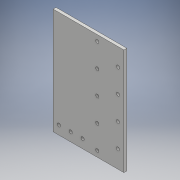
# Autodesk Inventor part: GanrtyPlatev2
Saved by Autodesk Inventor 2017 (Build 210142000, 142)
## iProperties
Created: 2017-03-07
Part Number: GanrtyPlatev2
Material: Generic
Document SubType Name: Modeling
Designer: umr
Density: 1 g/cm^3
Appearance: Default
Author: umr
Autodesk Inventor part; units mm, degrees
ref_plane "YZ Plane" through (0, 0, 0) normal (1, 0, 0) x (0, 1, 0)
ref_plane "XZ Plane" through (0, 0, 0) normal (0, 1, 0) x (-1, 0, 0)
ref_plane "XY Plane" through (0, 0, 0) normal (0, 0, 1) x (1, 0, 0)
sketch "Sketch1" plane through (0, 0, 0) normal (0, 1, 0) x (-1, 0, 0)
  line L0 (0, 0) -> (120, 0)
  line L1 (120, 0) -> (120, -180)
  line L2 (120, -180) -> (0, -180)
  line L3 (0, -180) -> (0, 0)
  dimension "d0" = 120
  dimension "d1" = 180
  constraints: 8 end point, 2 parallel, 1 horizontal, 1 perpendicular
  measures "d0" distance of L1.end L2.end
  measures "d1" distance of L0.end L1.end
extrude "Extrusion1" add sketch "Sketch1" along normal blind 5
sketch "Sketch2" plane through (0, 5, 0) normal (0, 1, 0) x (1, 0, 0)
  circle A0 centre (-45, 10) radius 2.75
  line L0 (-120, 0) -> (0, 0) projected
  line L1 (0, 0) -> (0, 180) projected
  circle A1 centre (-45, 50) radius 2.75
  circle A2 centre (-45, 90) radius 2.75
  circle A3 centre (-45, 130) radius 2.75
  circle A4 centre (-45, 170) radius 2.75
  circle A5 centre (-10, 30) radius 2.75
  circle A6 centre (-10, 70) radius 2.75
  circle A7 centre (-10, 110) radius 2.75
  circle A8 centre (-10, 150) radius 2.75
  dimension "d4" = 5.5
  dimension "d5" = 10
  dimension "d8" = 40
  dimension "d13" = 45
  dimension "d14" = 5.5
  dimension "d15" = 10
  dimension "d16" = 180
  dimension "d17" = 30
  dimension "d20" = 40
  constraints: 9 centre point, 2 vertical, 14 other
  measures "d4" diameter of A0
  measures "d5" distance from line of L0 A0.centre
  measures "d8" distance of A0.centre A1.centre
  measures "d13" distance from line of L1 A0.centre
  measures "d14" diameter of A5
  measures "d15" distance from line of L1 A5.centre
  measures "d16" distance of L0.end L1.end
  measures "d17" distance from line of L0 A5.centre
  measures "d20" distance of A5.centre A6.centre
extrude "Extrusion2" cut sketch "Sketch2" against normal blind 5
sketch "Sketch3" plane through (0, 5, 0) normal (0, 1, 0) x (1, 0, 0)
  circle A0 centre (-110, 165) radius 2.75
  line L0 (0, 180) -> (-120, 180) projected
  circle A1 centre (-90, 165) radius 2.75
  circle A2 centre (-70, 165) radius 2.75
  line L1 (-120, 180) -> (-120, 0) projected
  point P0 (0, 0)
  dimension "d27" = 5.5
  dimension "d28" = 15
  dimension "d31" = 20
  dimension "d38" = 10
  constraints: 3 centre point, 1 horizontal, 4 other
  measures "d27" diameter of A0
  measures "d28" distance from line of L0 A0.centre
  measures "d31" distance of A0.centre A1.centre
  measures "d38" distance from line of L1 A0.centre
extrude "Extrusion3" cut sketch "Sketch3" against normal blind 5
body "Solid1"
